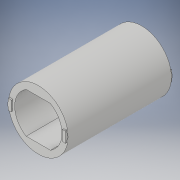
# Autodesk Inventor part: double recive corridor
Saved by Autodesk Inventor 2017 (Build 210142000, 142)
## iProperties
Created: 2018-03-04
Part Number: double recive corridor
Material: Generic
Document SubType Name: Modeling
Designer: Braxton
Density: 1 g/cm^3
Appearance: Default
Author: Braxton
Autodesk Inventor part; units mm, degrees
ref_plane "YZ Plane" through (0, 0, 0) normal (1, 0, 0) x (0, 1, 0)
ref_plane "XZ Plane" through (0, 0, 0) normal (0, 1, 0) x (-1, 0, 0)
ref_plane "XY Plane" through (0, 0, 0) normal (0, 0, 1) x (1, 0, 0)
sketch "Sketch1" plane through (0, 0, 0) normal (0, 0, 1) x (1, 0, 0)
  line L0 (-50.8, 84.6667) -> (50.8, 84.6667)
  line L1 (-50.8, -84.6667) -> (50.8, -84.6667)
  circle A0 centre (0, 0) radius 124.1375
  arc A1 (-50.8, 84.6667) -> (-50.8, -84.6667) centre (0, 0) ccw
  arc A2 (50.8, -84.6667) -> (50.8, 84.6667) centre (0, 0) ccw
  dimension "d0" = 169.3333
  dimension "d1" = 101.6
  constraints: 4 end point, 4 point on circle, 3 centre point, 2 coincident, 1 horizontal, 1 parallel
  measures "d0" distance between parallel lines of L1 L0
  measures "d1" distance of L0.start L0.end
extrude "corridor" add sketch "Sketch1" along normal blind 431.8
sketch "Sketch3" plane through (0, 0, 0) normal (0, 0, -1) x (-1, 0, 0)
  line L0 (0, 0) -> (118.4113, -23.1342)
  line L1 (0, 0) -> (118.4113, 23.1342)
  arc A0 (118.4113, -23.1342) -> (118.4113, 23.1342) centre (0, 0) ccw
  line L2 (107.95, 0) -> (120.65, 0)
  line L3 (120.65, 0) -> (107.95, 0)
  arc A1 (105.9469, -20.699) -> (105.9469, 20.699) centre (0, 0) ccw
  line L4 (-50.8, 84.6667) -> (50.8, 84.6667)
  line L5 (50.8, -84.6667) -> (-50.8, -84.6667)
  line L6 (0, 84.6667) -> (0, -84.6667) construction
  arc A2 (-50.8, 84.6667) -> (-50.8, -84.6667) centre (0, 0) ccw
  arc A3 (-105.9469, 20.699) -> (-105.9469, -20.699) centre (0, 0) ccw
  line L7 (0, 0) -> (-118.4113, -23.1342)
  arc A4 (-118.4113, 23.1342) -> (-118.4113, -23.1342) centre (0, 0) ccw
  line L8 (0, 0) -> (-118.4113, 23.1342)
  line L9 (-120.65, 0) -> (-107.95, 0)
  dimension "d20" = 11.055
  dimension "d21" = 11.055
  constraints: 20 end point, 14 point on circle, 5 centre point, 5 point on line, 4 symmetric about line, 3 coincident, 2 midpoint, 1 horizontal, 2 other
  measures "d20" angle of L9 L8
  measures "d21" angle of L9 L7
extrude "connection" add sketch "Sketch3" along normal blind 6.35 contours A1 L2 A0 L0 | L1 A0 L2 A1 | L7 A4 L9 A3 | A3 L9 A4 L8
ref_plane "mirror plane" through (0, 0, 215.9) normal (0, 0, 1) x (1, 0, 0)
mirror "Mirror connetion" about plane through (0, 0, 215.9) normal (0, 0, 1) of "connection"
equation "\"d21\" = d20"
body "Solid1"
